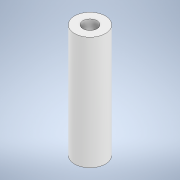
# Autodesk Inventor part: GenevaPin
Saved by Autodesk Inventor 2020.1 (Build 241239000, 239)
## iProperties
Created: 2019-11-10
Part Number: GenevaPin
Material: ABS Plastic
Document SubType Name: Modeling
Designer: Paul Lefeuvre
Density: 1.06 g/cm^3
Appearance: Smooth - White
Author: Paul Lefeuvre
Autodesk Inventor part; units mm, degrees
ref_plane "YZ Plane" through (0, 0, 0) normal (1, 0, 0) x (0, 1, 0)
ref_plane "XZ Plane" through (0, 0, 0) normal (0, 1, 0) x (-1, 0, 0)
ref_plane "XY Plane" through (0, 0, 0) normal (0, 0, 1) x (1, 0, 0)
sketch "Sketch1" plane through (0, 0, 0) normal (0, 1, 0) x (-1, 0, 0)
  circle A0 centre (0, 0) radius 3.91
  circle A1 centre (0, 0) radius 8.5
  line L0 (5.7735, 0) -> (2.8868, -5) construction
  line L1 (2.8868, -5) -> (-2.8868, -5) construction
  line L2 (-2.8868, -5) -> (-5.7735, 0) construction
  line L3 (-5.7735, 0) -> (-2.8868, 5) construction
  line L4 (-2.8868, 5) -> (2.8868, 5) construction
  line L5 (2.8868, 5) -> (5.7735, 0) construction
  line L6 (3.2332, -5.6) -> (6.4663, 0)
  line L7 (6.4663, 0) -> (3.2332, 5.6)
  line L8 (3.2332, 5.6) -> (-3.2332, 5.6)
  line L9 (-3.2332, 5.6) -> (-6.4663, 0)
  line L10 (-6.4663, 0) -> (-3.2332, -5.6)
  line L11 (-3.2332, -5.6) -> (3.2332, -5.6)
  dimension "d0" = 7.82
  dimension "d4" = 10
  dimension "d5" = 0.6
  dimension "d6" = 17
  constraints: 24 end point, 3 coincident, 2 centre point, 18 other
  measures "d0" diameter of A0
  measures "d4" distance of L4.end L0.end
  measures "d5" distance between parallel lines of L0 L6
  measures "d6" diameter of A1
extrude "Extrusion1" add sketch "Sketch1" along normal blind 62.6 contours A1 | L11 L10 L9 L8 L7 L6
extrude "Extrusion2" cut sketch "Sketch1" along normal blind 5.8 contours L11 L10 L9 L8 L7 L6
fillet "Fillet1" radius 0.5 6 edges at (-4.8497, 0, -2.8) (0, 0, -5.6) (4.8497, 0, -2.8) (4.8497, 0, 2.8) (0, 0, 5.6) (-4.8497, 0, 2.8)
body "Solid1"
